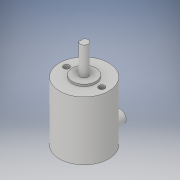
# Autodesk Inventor part: codeur_S25J
Saved by Autodesk Inventor 2019 (Build 230136000, 136)
## iProperties
Created: 2020-02-16
Part Number: codeur_S25J
Material: Generic
Document SubType Name: Modeling
Designer: franc
Density: 1 g/cm^3
Appearance: Default
Author: franc
Autodesk Inventor part; units mm, degrees
ref_plane "YZ Plane" through (0, 0, 0) normal (1, 0, 0) x (0, 1, 0)
ref_plane "XZ Plane" through (0, 0, 0) normal (0, 1, 0) x (-1, 0, 0)
sketch "Esquisse1" plane through (0, 0, 0) normal (0, 1, 0) x (-1, 0, 0)
  circle A0 centre (0, 0) radius 12.5
  dimension "d0" = 25
  constraints: 1 centre point, 1 coincident
  measures "d0" diameter of A0
extrude "Extrusion1" add sketch "Esquisse1" along normal blind 30
sketch "Esquisse2" plane through (0, 30, 0) normal (0, 1, 0) x (1, 0, 0)
  circle A0 centre (0, 0) radius 6
  dimension "d3" = 12
  constraints: 1 centre point, 1 coincident
  measures "d3" diameter of A0
extrude "Extrusion2" add sketch "Esquisse2" along normal blind 1
sketch "Esquisse3" plane through (0, 31, 0) normal (0, 1, 0) x (1, 0, 0)
  circle A0 centre (0, 0) radius 2
  dimension "d6" = 4
  constraints: 1 centre point, 1 coincident
  measures "d6" diameter of A0
extrude "Extrusion3" add sketch "Esquisse3" along normal blind 14.5
sketch "Esquisse4" plane through (0, 45.5, 0) normal (0, 1, 0) x (1, 0, 0)
  circle A0 centre (0, 0) radius 2 projected
  line L0 (-1.5, -1.3229) -> (-1.5, 1.3229)
  dimension "d9" = 0.5
  constraints: 2 end point, 2 point on circle, 1 vertical
  measures "d9" distance edge to line of A0 L0
extrude "Extrusion4" cut sketch "Esquisse4" against normal blind 7 contours L0 A0 picked at (-1.5908, -0.3089)
ref_plane "Plan de construction1" through (0, 0, -12.5) normal (0, 0, 1) x (1, 0, 0)
sketch "Esquisse5" plane through (0, 0, -12.5) normal (0, 0, 1) x (1, 0, 0)
  circle A0 centre (0, 3.5) radius 3.5
  point P0 (0, 0)
  dimension "d12" = 3.5
  dimension "d13" = 7
  constraints: 1 centre point
  measures "d12" distance of point (0, 0) A0.centre
  measures "d13" diameter of A0
extrude "Extrusion5" add sketch "Esquisse5" along normal mid plane 2
sketch "Esquisse6" plane through (0, 3.5, -13.5) normal (0, 0, -1) x (-1, 0, 0)
  circle A0 centre (0, 0) radius 3
  point P0 (0, -3.5)
  dimension "d16" = 6
  constraints: 1 centre point
  measures "d16" diameter of A0
extrude "Extrusion6" add sketch "Esquisse6" along normal blind 5
sketch "Esquisse7" plane through (0, 30, 0) normal (0, 1, 0) x (1, 0, 0)
  circle A0 centre (-9, 0) radius 1.5
  circle A1 centre (9, 0) radius 1.5
  point P0 (0, 0)
  dimension "d19" = 3
  dimension "d20" = 3
  dimension "d21" = 9
  dimension "d22" = 9
  constraints: 2 centre point
  measures "d19" diameter of A0
  measures "d20" diameter of A1
  measures "d21" distance of point (0, 0) A0.centre
  measures "d22" distance of point (0, 0) A1.centre
extrude "Extrusion7" cut sketch "Esquisse7" against normal blind 5
